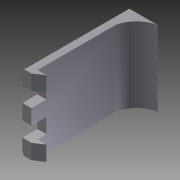
# Autodesk Inventor part: parteA
Saved by Autodesk Inventor 2012 (Build 160160000, 160)
## iProperties
Created: 2013-01-02
Part Number: parteA
Material: Default
Document SubType Name: Modeling
Designer: asimov
Density: 1 g/cm^3
Author: asimov
Autodesk Inventor part; units mm, degrees
ref_plane "YZ Plane" through (0, 0, 0) normal (1, 0, 0) x (0, 1, 0)
ref_plane "XZ Plane" through (0, 0, 0) normal (0, 1, 0) x (-1, 0, 0)
ref_plane "XY Plane" through (0, 0, 0) normal (0, 0, 1) x (1, 0, 0)
sketch "Sketch1" plane through (0, 0, 0) normal (0, 0, 1) x (1, 0, 0)
  line L0 (0, 0) -> (0, 35)
  line L1 (0, 35) -> (3, 35)
  line L2 (3, 28) -> (3, 2)
  line L3 (3, 0) -> (0, 0)
  line L4 (3, 2) -> (6, 2)
  line L5 (6, 2) -> (3, 0)
  line L6 (10, 35) -> (3, 35)
  arc A0 (10, 35) -> (3, 28) centre (11.8151, 26.1849) ccw
  dimension "d7" = 9
  dimension "d8" = 3
  dimension "d9" = 7
  dimension "d10" = 7
  constraints: 14 end point, 3 perpendicular, 2 point on circle, 1 centre point, 1 parallel, 1 vertical
  measures "d7" radius of A0
  measures "d8" distance of L3.start L0.start
  measures "d9" distance of L2.start L1.end
  measures "d10" distance of L6.start L1.end
extrude "Extrusion1" add sketch "Sketch1" along normal blind 25
fillet "Fillet1" radius 1 1 edges at (0, 17.5, 25)
fillet "Fillet2" radius 1 1 edges at (0, 17.5, 0)
sketch "Sketch2" plane through (3, 0, 0) normal (0, -1, 0) x (1, 0, 0)
  line L0 (-3, 1) -> (-3, 24) projected
  line L1 (0, 5) -> (-3, 5)
  line L2 (-3, 5) -> (-3, 10)
  line L3 (-3, 10) -> (0, 10)
  line L4 (0, 15) -> (-3, 15)
  line L5 (0, 20) -> (-3, 20)
  line L6 (-3, 15) -> (-3, 20)
  line L7 (3.0852, 20) -> (0, 20)
  line L8 (3.0852, 20) -> (3.0852, 15)
  line L9 (3.0852, 15) -> (-1, 15)
  line L10 (0, 10) -> (1.0426, 10)
  line L11 (1.0426, 10) -> (3.0852, 10)
  line L12 (3.0852, 10) -> (3.0852, 5)
  line L13 (3.0852, 5) -> (0, 5)
  point P0 (-3, 0)
  dimension "d17" = 5
  constraints: 26 end point, 5 point on line, 3 collinear, 3 perpendicular, 2 parallel
  measures "d17" distance of L1.end L2.end
extrude "Extrusion2" cut sketch "Sketch2" against normal blind 5
sketch "Sketch3" plane through (3, 2, 10) normal (0, 1, 0) x (1, 0, 0)
  line L0 (3, 0) -> (0, 0) projected
  line L1 (0, -5) -> (3, -5) projected
  line L2 (3, 0) -> (3, -5) projected
  line L3 (0, -5) -> (0, 0)
  line L4 (3, 0) -> (0, 0)
  line L5 (3, 0) -> (3, -5)
  line L6 (3, -5) -> (0, -5)
  point P0 (-3, 10)
  constraints: 8 end point, 2 equal length, 2 perpendicular
extrude "Extrusion3" cut sketch "Sketch3" against normal blind 5
body "Solid1"
